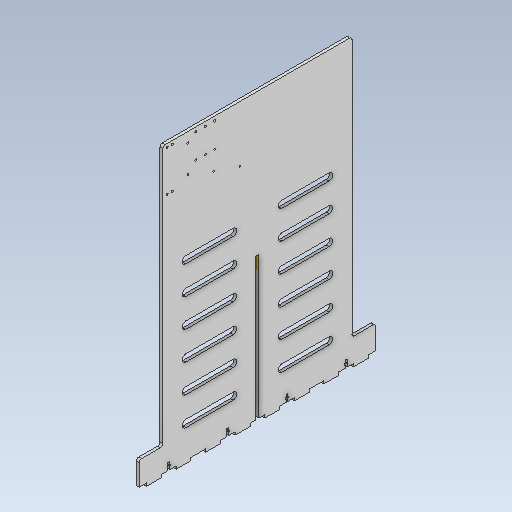
# Autodesk Inventor part: Korpus 2
Saved by Autodesk Inventor 2021.1 (Build 251245010, 245A)
## iProperties
Created: 2023-03-13
Part Number: Korpus 2
Material: Типовые
Document SubType Name: Modeling
Designer: User
Density: 1 g/cm^3
Appearance: По умолчанию
Author: User
Autodesk Inventor part; units mm, degrees
ref_plane "YZ Plane" through (0, 0, 0) normal (1, 0, 0) x (0, 1, 0)
ref_plane "XZ Plane" through (0, 0, 0) normal (0, 1, 0) x (-1, 0, 0)
ref_plane "XY Plane" through (0, 0, 0) normal (0, 0, 1) x (1, 0, 0)
ref_plane "РабПлоскость1" through (105.5444, -154.3829, -245.2468) normal (1, 0, 0) x (0, 1, 0)
sketch "Эскиз1" plane through (105.5444, -154.3829, -245.2468) normal (1, 0, 0) x (0, 1, 0)
  line L0 (-283.5683, 0) -> (167.3606, 0) construction
  line L1 (16.4317, 0) -> (316.4317, 0) construction
  line L2 (16.4317, 6) -> (316.4317, 6) construction
  line L3 (-283.5683, 6) -> (167.3606, 6) construction
  line L4 (316.4317, 6) -> (316.4317, 0) construction
  line L5 (316.4317, 198) -> (316.4317, -192)
  line L6 (-283.5683, 268.625) -> (-283.5683, 237.375) construction
  line L7 (-283.5683, 237.375) -> (-289.5683, 237.375)
  line L8 (-289.5683, 237.375) -> (-289.5683, 206.125)
  line L9 (-289.5683, 206.125) -> (-283.5683, 206.125)
  line L10 (-283.5683, 206.125) -> (-283.5683, 174.875)
  line L11 (-283.5683, 174.875) -> (-289.5683, 174.875)
  line L12 (-289.5683, 174.875) -> (-289.5683, 143.625)
  line L13 (-289.5683, 143.625) -> (-283.5683, 143.625)
  line L14 (-283.5683, 143.625) -> (-283.5683, 112.375)
  line L15 (-283.5683, 112.375) -> (-289.5683, 112.375)
  line L16 (-289.5683, 112.375) -> (-289.5683, 81.125)
  line L17 (-289.5683, 81.125) -> (-283.5683, 81.125)
  line L18 (-283.5683, 81.125) -> (-283.5683, 49.875)
  line L19 (-283.5683, 49.875) -> (-289.5683, 49.875)
  line L20 (-289.5683, 49.875) -> (-289.5683, 18.625)
  line L21 (-289.5683, 18.625) -> (-283.5683, 18.625)
  line L22 (-283.5683, 18.625) -> (-283.5683, -12.625) construction
  line L23 (-283.5683, -12.625) -> (-289.5683, -12.625)
  line L24 (-289.5683, -12.625) -> (-289.5683, -43.875)
  line L25 (-289.5683, -43.875) -> (-283.5683, -43.875)
  line L26 (-283.5683, -43.875) -> (-283.5683, -75.125)
  line L27 (-283.5683, -75.125) -> (-289.5683, -75.125)
  line L28 (-289.5683, -75.125) -> (-289.5683, -106.375)
  line L29 (-289.5683, -106.375) -> (-283.5683, -106.375)
  line L30 (-283.5683, -106.375) -> (-283.5683, -137.625)
  line L31 (-283.5683, -137.625) -> (-289.5683, -137.625)
  line L32 (-289.5683, -137.625) -> (-289.5683, -168.875)
  line L33 (-289.5683, -168.875) -> (-283.5683, -168.875)
  line L34 (-283.5683, -168.875) -> (-283.5683, -200.125)
  line L35 (-283.5683, -200.125) -> (-289.5683, -200.125)
  line L36 (-289.5683, -200.125) -> (-289.5683, -231.375)
  line L37 (-289.5683, -231.375) -> (-283.5683, -231.375)
  line L38 (-283.5683, -231.375) -> (-283.5683, -262.625) construction
  line L39 (-283.5683, -247) -> (-283.5683, -231.375)
  line L40 (-283.5683, 237.375) -> (-283.5683, 253)
  line L41 (-283.5683, 253) -> (-238.5683, 253)
  line L42 (-283.5683, -247) -> (-238.5683, -247)
  line L43 (-289.5683, 0) -> (-283.5683, 0) construction
  line L44 (-283.5683, 6) -> (-283.5683, 0) construction
  line L45 (311.4317, 203) -> (-228.5683, 203)
  line L46 (-233.5683, 208) -> (-233.5683, 248)
  line L47 (311.4317, -197) -> (-228.5683, -197)
  line L48 (-233.5683, -202) -> (-233.5683, -242)
  arc A0 (-233.5683, 248) -> (-238.5683, 253) centre (-238.5683, 248) ccw
  arc A1 (-233.5683, 208) -> (-228.5683, 203) centre (-228.5683, 208) ccw
  arc A2 (316.4317, 198) -> (311.4317, 203) centre (311.4317, 198) ccw
  arc A3 (311.4317, -197) -> (316.4317, -192) centre (311.4317, -192) ccw
  arc A4 (-228.5683, -197) -> (-233.5683, -202) centre (-228.5683, -202) ccw
  arc A5 (-238.5683, -247) -> (-233.5683, -242) centre (-238.5683, -242) ccw
  line L49 (76.4317, 0) -> (91.4317, 0) projected
  line L50 (76.4317, 6) -> (91.4317, 6) projected
  line L51 (16.4317, 0) -> (31.4317, 0) projected
  line L52 (16.4317, 6) -> (31.4317, 6) projected
  line L53 (-43.5683, 0) -> (-28.5683, 0) projected
  line L54 (-43.5683, 6) -> (-28.5683, 6) projected
  line L55 (-103.5683, 0) -> (-88.5683, 0) projected
  line L56 (-103.5683, 6) -> (-88.5683, 6) projected
  line L57 (-163.5683, 0) -> (-148.5683, 0) projected
  line L58 (-163.5683, 6) -> (-148.5683, 6) projected
  line L59 (-223.5683, 0) -> (-208.5683, 0) projected
  line L60 (-223.5683, 6) -> (-208.5683, 6) projected
  arc A6 (91.4317, 154.5) -> (76.4317, 154.5) centre (83.9317, 154.5) ccw
  arc A7 (31.4317, 154.5) -> (16.4317, 154.5) centre (23.9317, 154.5) ccw
  arc A8 (-28.5683, 154.5) -> (-43.5683, 154.5) centre (-36.0683, 154.5) ccw
  arc A9 (-88.5683, 154.5) -> (-103.5683, 154.5) centre (-96.0683, 154.5) ccw
  arc A10 (-148.5683, 154.5) -> (-163.5683, 154.5) centre (-156.0683, 154.5) ccw
  arc A11 (-208.5683, 154.5) -> (-223.5683, 154.5) centre (-216.0683, 154.5) ccw
  arc A12 (76.4317, 54.5) -> (91.4317, 54.5) centre (83.9317, 54.5) ccw
  arc A13 (16.4317, 54.5) -> (31.4317, 54.5) centre (23.9317, 54.5) ccw
  arc A14 (-43.5683, 54.5) -> (-28.5683, 54.5) centre (-36.0683, 54.5) ccw
  arc A15 (-103.5683, 54.5) -> (-88.5683, 54.5) centre (-96.0683, 54.5) ccw
  arc A16 (-163.5683, 54.5) -> (-148.5683, 54.5) centre (-156.0683, 54.5) ccw
  arc A17 (-223.5683, 54.5) -> (-208.5683, 54.5) centre (-216.0683, 54.5) ccw
  line L61 (91.4317, 154.5) -> (91.4317, 54.5)
  line L62 (76.4317, 154.5) -> (76.4317, 54.5)
  line L63 (31.4317, 154.5) -> (31.4317, 54.5)
  line L64 (16.4317, 154.5) -> (16.4317, 54.5)
  line L65 (-28.5683, 154.5) -> (-28.5683, 54.5)
  line L66 (-43.5683, 154.5) -> (-43.5683, 54.5)
  line L67 (-88.5683, 154.5) -> (-88.5683, 54.5)
  line L68 (-103.5683, 154.5) -> (-103.5683, 54.5)
  line L69 (-148.5683, 154.5) -> (-148.5683, 54.5)
  line L70 (-163.5683, 154.5) -> (-163.5683, 54.5)
  line L71 (-208.5683, 154.5) -> (-208.5683, 54.5)
  line L72 (-223.5683, 154.5) -> (-223.5683, 54.5)
  line L73 (83.9317, 154.5) -> (83.9317, 203) construction
  line L74 (83.9317, 54.5) -> (83.9317, 6) construction
  line L75 (23.9317, 54.5) -> (23.9317, 6) construction
  line L76 (23.9317, 154.5) -> (23.9317, 203) construction
  line L77 (-36.0683, 154.5) -> (-36.0683, 203) construction
  line L78 (-36.0683, 54.5) -> (-36.0683, 6) construction
  line L79 (-96.0683, 54.5) -> (-96.0683, 6) construction
  line L80 (-96.0683, 154.5) -> (-96.0683, 203) construction
  line L81 (-156.0683, 154.5) -> (-156.0683, 203) construction
  line L82 (-156.0683, 54.5) -> (-156.0683, 6) construction
  line L83 (-216.0683, 54.5) -> (-216.0683, 6) construction
  line L84 (-216.0683, 154.5) -> (-216.0683, 203) construction
  arc A18 (76.4317, -148.5) -> (91.4317, -148.5) centre (83.9317, -148.5) ccw
  arc A19 (16.4317, -148.5) -> (31.4317, -148.5) centre (23.9317, -148.5) ccw
  arc A20 (-43.5683, -148.5) -> (-28.5683, -148.5) centre (-36.0683, -148.5) ccw
  arc A21 (-103.5683, -148.5) -> (-88.5683, -148.5) centre (-96.0683, -148.5) ccw
  arc A22 (-163.5683, -148.5) -> (-148.5683, -148.5) centre (-156.0683, -148.5) ccw
  arc A23 (-223.5683, -148.5) -> (-208.5683, -148.5) centre (-216.0683, -148.5) ccw
  arc A24 (91.4317, -48.5) -> (76.4317, -48.5) centre (83.9317, -48.5) ccw
  arc A25 (31.4317, -48.5) -> (16.4317, -48.5) centre (23.9317, -48.5) ccw
  arc A26 (-28.5683, -48.5) -> (-43.5683, -48.5) centre (-36.0683, -48.5) ccw
  arc A27 (-88.5683, -48.5) -> (-103.5683, -48.5) centre (-96.0683, -48.5) ccw
  arc A28 (-148.5683, -48.5) -> (-163.5683, -48.5) centre (-156.0683, -48.5) ccw
  arc A29 (-208.5683, -48.5) -> (-223.5683, -48.5) centre (-216.0683, -48.5) ccw
  line L85 (91.4317, -148.5) -> (91.4317, -48.5)
  line L86 (76.4317, -148.5) -> (76.4317, -48.5)
  line L87 (31.4317, -148.5) -> (31.4317, -48.5)
  line L88 (16.4317, -148.5) -> (16.4317, -48.5)
  line L89 (-28.5683, -148.5) -> (-28.5683, -48.5)
  line L90 (-43.5683, -148.5) -> (-43.5683, -48.5)
  line L91 (-88.5683, -148.5) -> (-88.5683, -48.5)
  line L92 (-103.5683, -148.5) -> (-103.5683, -48.5)
  line L93 (-148.5683, -148.5) -> (-148.5683, -48.5)
  line L94 (-163.5683, -148.5) -> (-163.5683, -48.5)
  line L95 (-208.5683, -148.5) -> (-208.5683, -48.5)
  line L96 (-223.5683, -148.5) -> (-223.5683, -48.5)
  line L97 (316.4317, 3) -> (-283.5683, 3) construction
  line L98 (16.4317, 6) -> (16.4317, 0)
  line L99 (16.4317, 6) -> (-283.5683, 6)
  line L100 (-283.5683, 0) -> (16.4317, 0)
  line L101 (83.9317, 0) -> (83.9317, -48.5) construction
  line L102 (83.9317, -148.5) -> (83.9317, -197) construction
  line L103 (23.9317, -148.5) -> (23.9317, -197) construction
  line L104 (23.9317, -48.5) -> (23.9317, 0) construction
  line L105 (-36.0683, 0) -> (-36.0683, -48.5) construction
  line L106 (-36.0683, -148.5) -> (-36.0683, -197) construction
  line L107 (-96.0683, -148.5) -> (-96.0683, -197) construction
  line L108 (-96.0683, -48.5) -> (-96.0683, 0) construction
  line L109 (-156.0683, -48.5) -> (-156.0683, 0) construction
  line L110 (-156.0683, -148.5) -> (-156.0683, -197) construction
  line L111 (-216.0683, -148.5) -> (-216.0683, -197) construction
  line L112 (-216.0683, -48.5) -> (-216.0683, 0) construction
  line L113 (-283.5683, 18.625) -> (-283.5683, 6)
  line L114 (-283.5683, 0) -> (-283.5683, -12.625)
  point P0 (154.3829, 245.2468)
  point P1 (316.4317, 203)
  point P2 (316.4317, -197)
  point P3 (-233.5683, 253)
  point P4 (-233.5683, -197)
  point P5 (-233.5683, -269.5287)
  point P6 (91.4317, 104.5)
  point P7 (76.4317, 104.5)
  point P8 (31.4317, 104.5)
  point P9 (16.4317, 104.5)
  point P10 (-28.5683, 104.5)
  point P11 (-43.5683, 104.5)
  point P12 (-88.5683, 104.5)
  point P13 (-103.5683, 104.5)
  point P14 (-148.5683, 104.5)
  point P15 (-163.5683, 104.5)
  point P16 (-208.5683, 104.5)
  point P17 (-223.5683, 104.5)
  point P18 (76.5, -98.5)
  point P19 (61.5, -98.5)
  point P20 (16.5, -98.5)
  point P21 (1.5, -98.5)
  point P22 (-43.5, -98.5)
  point P23 (-58.5, -98.5)
  point P24 (-103.5, -98.5)
  point P25 (-118.5, -98.5)
  point P26 (-163.5, -98.5)
  point P27 (-178.5, -98.5)
  point P28 (-223.5, -98.5)
  point P29 (-238.5, -98.5)
  point P30 (16.4317, 3)
  point P31 (-223.5683, 6)
  point P32 (-208.5683, 6)
  point P33 (-163.5683, 6)
  point P34 (-148.5683, 6)
  point P35 (-103.5683, 6)
  point P36 (-88.5683, 6)
  point P37 (-43.5683, 6)
  point P38 (-28.5683, 6)
  point P39 (-28.5683, 0)
  point P40 (-43.5683, 0)
  point P41 (-88.5683, 0)
  point P42 (-103.5683, 0)
  point P43 (-148.5683, 0)
  point P44 (-163.5683, 0)
  point P45 (-208.5683, 0)
  point P46 (-223.5683, 0)
  dimension "d0" = 400
  dimension "d1" = 500
  dimension "d2" = 6
  dimension "d3" = 50
  dimension "d4" = 5
  dimension "d5" = 100
  dimension "d8" = 6
  constraints: 168 end point, 60 point on circle, 40 point on line, 37 vertical, 32 tangent, 30 centre point, 30 midpoint, 25 parallel, 25 vertical alignment, 19 perpendicular, 16 collinear, 5 equal radius, 4 horizontal, 87 other
  measures "d0" distance of point (316.432, 203) point (316.432, -197)
  measures "d1" distance between parallel lines of L42 L41
  measures "d2" distance of L36.end L37.end
  measures "d3" distance of L40.end point (-233.568, 253)
  measures "d4" radius of A0
  measures "d5" distance of L61.start L61.end
  measures "d8" distance of L98.start L98.end
extrude "Корпус" add sketch "Эскиз1" along normal blind 6
sketch "Эскиз2" plane through (105.5444, -154.3829, -245.2468) normal (-1, 0, 0) x (0, 0, 1)
  circle A0 centre (-188, 309.4317) radius 2.1 construction
  circle A1 centre (-177, 309.4317) radius 2.1 construction
  circle A2 centre (-188, 223.4317) radius 2.1 construction
  circle A3 centre (-177, 223.4317) radius 2.1 construction
  line L0 (-192, 316.4317) -> (198, 316.4317) construction
  line L1 (-197, -228.5683) -> (-197, 311.4317) construction
  circle A4 centre (-144, 295.4317) radius 2.1 construction
  circle A5 centre (-144, 237.4317) radius 2.1 construction
  line L2 (-144, 295.4317) -> (-144, 309.4317) construction
  line L3 (-144, 237.4317) -> (-144, 223.4317) construction
  circle A6 centre (-127.2, 307.6167) radius 2.1 construction
  circle A7 centre (-127.2, 255.7467) radius 2.1 construction
  circle A8 centre (-107.2, 307.6167) radius 2.1 construction
  circle A9 centre (-107.2, 255.7467) radius 2.1 construction
  circle A10 centre (-87.2, 307.6167) radius 2.1 construction
  circle A11 centre (-87.2, 255.7467) radius 2.1 construction
  line L4 (-127.2, 307.6167) -> (-107.2, 307.6167) construction
  line L5 (-107.2, 307.6167) -> (-87.2, 307.6167) construction
  circle A12 centre (-34.5, 197.4317) radius 1.6 construction
  circle A13 centre (-89.5, 216.4317) radius 1.6 construction
  line L6 (3, 316.4317) -> (3, 241.6574) construction
  circle A14 centre (194, 309.4317) radius 2.1
  circle A15 centre (183, 309.4317) radius 2.1
  circle A16 centre (194, 223.4317) radius 2.1
  circle A17 centre (183, 223.4317) radius 2.1
  circle A18 centre (150, 295.4317) radius 2.1
  circle A19 centre (150, 237.4317) radius 2.1
  circle A20 centre (133.2, 307.6167) radius 2.1
  circle A21 centre (133.2, 255.7467) radius 2.1
  circle A22 centre (113.2, 307.6167) radius 2.1
  circle A23 centre (113.2, 255.7467) radius 2.1
  circle A24 centre (93.2, 307.6167) radius 2.1
  circle A25 centre (93.2, 255.7467) radius 2.1
  circle A26 centre (40.5, 197.4317) radius 1.6
  circle A27 centre (95.5, 216.4317) radius 1.6
  point P0 (245.2468, 154.3829)
  dimension "d9" = 4.2
  dimension "d10" = 7
  dimension "d11" = 20
  dimension "d12" = 9
  dimension "d13" = 93
  dimension "d14" = 21
  dimension "d15" = 53
  dimension "d16" = 69.8
  dimension "d17" = 8.815
  dimension "d18" = 60.685
  dimension "d19" = 89.8
  dimension "d20" = 162.5
  dimension "d21" = 107.5
  dimension "d22" = 100
  dimension "d23" = 119
  dimension "d24" = 3.2
  constraints: 28 centre point, 14 symmetric about line, 12 equal radius, 10 end point, 8 horizontal alignment, 6 vertical alignment, 3 collinear, 3 vertical, 1 horizontal, 1 midpoint, 14 other
  measures "d9" diameter of A0
  measures "d10" distance from line of L0 A1.centre
  measures "d11" distance from line of L1 A1.centre
  measures "d12" distance from line of L1 A0.centre
  measures "d13" distance from line of A3.centre L0
  measures "d14" distance from line of L0 L2.start
  measures "d15" distance from line of L1 L2.start
  measures "d16" distance from line of L1 A7.centre
  measures "d17" distance from line of L0 L4.start
  measures "d18" distance from line of L0 A7.centre
  measures "d19" distance from line of L1 A9.centre
  measures "d20" distance from line of L1 A12.centre
  measures "d21" distance from line of L1 A13.centre
  measures "d22" distance from line of L0 A13.centre
  measures "d23" distance from line of L0 A12.centre
  measures "d24" diameter of A12
extrude "Отверстия" cut sketch "Эскиз2" against normal blind 6
sketch "Эскиз3" plane through (111.5444, -154.3829, -245.2468) normal (1, 0, 0) x (0, 0, -1)
  line L0 (-192.5, -283.5683) -> (-192.5, -277.6183)
  line L1 (-192.5, -277.6183) -> (-193.9, -277.6183)
  line L2 (-193.9, -277.6183) -> (-193.9, -274.5183)
  line L3 (-193.9, -274.5183) -> (-192.5, -274.5183)
  line L4 (-192.5, -274.5183) -> (-192.5, -268.5683)
  line L5 (-192.5, -268.5683) -> (-188.5, -268.5683)
  line L6 (-188.5, -268.5683) -> (-188.5, -274.5183)
  line L7 (-188.5, -274.5183) -> (-187.1, -274.5183)
  line L8 (-187.1, -274.5183) -> (-187.1, -277.6183)
  line L9 (-187.1, -277.6183) -> (-188.5, -277.6183)
  line L10 (-188.5, -277.6183) -> (-188.5, -283.5683)
  line L11 (-192.5, -283.5683) -> (-188.5, -283.5683)
  line L12 (-67.5, -283.5683) -> (-67.5, -277.6183)
  line L13 (-67.5, -277.6183) -> (-68.9, -277.6183)
  line L14 (-68.9, -277.6183) -> (-68.9, -274.5183)
  line L15 (-68.9, -274.5183) -> (-67.5, -274.5183)
  line L16 (-67.5, -274.5183) -> (-67.5, -268.5683)
  line L17 (-67.5, -268.5683) -> (-63.5, -268.5683)
  line L18 (-63.5, -268.5683) -> (-63.5, -274.5183)
  line L19 (-63.5, -274.5183) -> (-62.1, -274.5183)
  line L20 (-62.1, -274.5183) -> (-62.1, -277.6183)
  line L21 (-62.1, -277.6183) -> (-63.5, -277.6183)
  line L22 (-63.5, -277.6183) -> (-63.5, -283.5683)
  line L23 (-67.5, -283.5683) -> (-63.5, -283.5683)
  line L24 (57.5, -283.5683) -> (57.5, -277.6183)
  line L25 (57.5, -277.6183) -> (56.1, -277.6183)
  line L26 (56.1, -277.6183) -> (56.1, -274.5183)
  line L27 (56.1, -274.5183) -> (57.5, -274.5183)
  line L28 (57.5, -274.5183) -> (57.5, -268.5683)
  line L29 (57.5, -268.5683) -> (61.5, -268.5683)
  line L30 (61.5, -268.5683) -> (61.5, -274.5183)
  line L31 (61.5, -274.5183) -> (62.9, -274.5183)
  line L32 (62.9, -274.5183) -> (62.9, -277.6183)
  line L33 (62.9, -277.6183) -> (61.5, -277.6183)
  line L34 (61.5, -277.6183) -> (61.5, -283.5683)
  line L35 (57.5, -283.5683) -> (61.5, -283.5683)
  line L36 (182.5, -283.5683) -> (182.5, -277.6183)
  line L37 (182.5, -277.6183) -> (181.1, -277.6183)
  line L38 (181.1, -277.6183) -> (181.1, -274.5183)
  line L39 (181.1, -274.5183) -> (182.5, -274.5183)
  line L40 (182.5, -274.5183) -> (182.5, -268.5683)
  line L41 (182.5, -268.5683) -> (186.5, -268.5683)
  line L42 (186.5, -268.5683) -> (186.5, -274.5183)
  line L43 (186.5, -274.5183) -> (187.9, -274.5183)
  line L44 (187.9, -274.5183) -> (187.9, -277.6183)
  line L45 (187.9, -277.6183) -> (186.5, -277.6183)
  line L46 (186.5, -277.6183) -> (186.5, -283.5683)
  line L47 (182.5, -283.5683) -> (186.5, -283.5683)
  line L48 (-192.5, -289.5683) -> (-192.5, -283.5683) construction
  line L49 (-188.5, -289.5683) -> (-188.5, -283.5683) construction
  line L50 (-188.5, -289.5683) -> (-188.5, -283.5683) construction
  line L51 (-192.5, -289.5683) -> (-192.5, -283.5683) construction
  point P0 (-245.2468, 154.3829)
  dimension "d32" = 125
  dimension "d39" = 15
  dimension "d40" = 6.8
  dimension "d41" = 3.1
  constraints: 104 end point, 28 point on line, 7 perpendicular, 5 vertical, 3 collinear, 2 coincident, 1 horizontal, 75 other
  measures "d32" distance of L0.start L12.start
  measures "d39" distance between parallel lines of L11 L5
  measures "d40" distance between parallel lines of L8 L2
  measures "d41" distance between parallel lines of L7 L9
extrude "Пазы" cut sketch "Эскиз3" against normal blind 6
equation "\"d5\" = 0.25 * d0"
equation "\"d8\" = d2"
equation "\"d6\" = d2"
equation "\"d25\" = d2"
equation "\"d32\" = 0.25 * d1"
equation "\"d37\" = d2"
